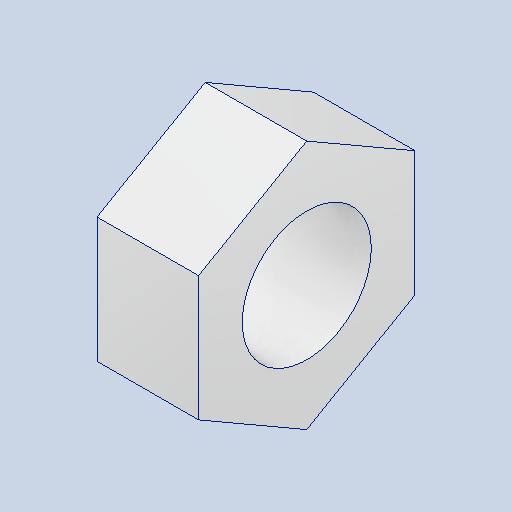
# Autodesk Inventor part: 4min-nut
Saved by Autodesk Inventor 2024.1 (Build 281209000, 209)
## iProperties
Created: 2023-09-27
Part Number: 4min-nut
Material: アルミニウム 6061
Document SubType Name: Modeling
Designer: haruy
Density: 2.7 g/cm^3
Appearance: アルミニウム - フラット
Author: haruy
Autodesk Inventor part; units mm, degrees
ref_plane "YZ Plane" through (0, 0, 0) normal (1, 0, 0) x (0, 1, 0)
ref_plane "XZ Plane" through (0, 0, 0) normal (0, 1, 0) x (-1, 0, 0)
ref_plane "XY Plane" through (0, 0, 0) normal (0, 0, 1) x (1, 0, 0)
sketch "スケッチ1" plane through (0, 0, 0) normal (1, 0, 0) x (0, 1, 0)
  circle A0 centre (0, 0) radius 2
  line L0 (3.875, 0) -> (1.9375, 3.3558)
  line L1 (1.9375, 3.3558) -> (-1.9375, 3.3558)
  line L2 (-1.9375, 3.3558) -> (-3.875, 0)
  line L3 (-3.875, 0) -> (-1.9375, -3.3558)
  line L4 (-1.9375, -3.3558) -> (1.9375, -3.3558)
  line L5 (1.9375, -3.3558) -> (3.875, 0)
  dimension "d0" = 4
  dimension "d1" = 3.875
  dimension "d4" = 360
  constraints: 12 end point, 3 parallel, 1 centre point, 1 coincident, 1 horizontal, 1 point on line, 7 other
  measures "d0" diameter of A0
  measures "d1" distance of point (0, 0) L0.start
extrude "押し出し1" add sketch "スケッチ1" along normal blind 3.15
